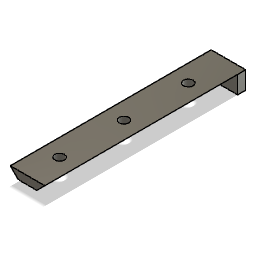
blind-joint-drill-guide-10mm-and-3z v3 (Autodesk Fusion 360 design; units mm, degrees)
Autodesk Fusion 360 part; units mm, degrees
sketch "Sketch1" plane through (0, 0, 0) normal (0, 0, 1) x (1, 0, 0)
  line L0 (-2.875, 0) -> (2.875, 0)
  line L1 (-5.375, 2.5) -> (5.375, 2.5)
  line L2 (-5.375, 2.5) -> (-2.875, 0)
  line L3 (5.375, 2.5) -> (2.875, 0)
  line L4 (0, 7.9451) -> (0, -6.0549)
  dimension "d1" = 5.75
  dimension "d2" = 10.75
  dimension "d3" = 2.5
  constraint horizontal L0
  constraint horizontal L1
  constraint vertical L4
  constraint symmetric L1.start L1.end L4
  constraint symmetric L0.start L0.end L4
  constraint vertical origin L4.end
  constraint horizontal origin L0.start
  measures "d1" distance of L0.start L0.end
  measures "d2" distance of L1.start L1.end
  measures "d3" vertical distance of L0.start L1.start
extrude "Extrude1" add sketch "Sketch1" along normal blind 60
sketch "Sketch2" plane through (0, 0, 0) normal (0, 0, -1) x (-1, 0, 0)
  line L0 (2.875, 0) -> (5.375, 2.5)
  line L1 (5.375, 2.5) -> (-5.375, 2.5)
  line L2 (-5.375, 2.5) -> (-2.875, 0)
  line L3 (-2.875, 0) -> (2.875, 0)
  line L4 (-5.375, 2.5) -> (5.375, 2.5)
  line L5 (5.375, 2.5) -> (5.375, -3)
  line L6 (5.375, -3) -> (-5.375, -3)
  line L7 (-5.375, -3) -> (-5.375, 2.5)
  dimension "d6" = 10.75
  dimension "d7" = 5.5
  constraint horizontal L4
  constraint vertical L5
  constraint horizontal L6
  constraint vertical L7
  constraint coincident L1.end L2.start
  measures "d6" distance of L1.end L0.end
  measures "d7" distance of L1.end L6.end
extrude "Extrude2" add sketch "Sketch2" along normal blind 2.5
sketch "Sketch3" plane through (0, 0, 0) normal (0, -1, 0) x (1, 0, 0)
  line L0 (-2.875, 0) -> (2.875, 0)
  line L1 (2.875, 0) -> (2.875, 60)
  line L2 (2.875, 60) -> (-2.875, 60)
  line L3 (-2.875, 60) -> (-2.875, 0)
  circle A0 centre (0, 10) radius 1.5
  circle A1 centre (0, 30) radius 1.5
  circle A2 centre (0, 50) radius 1.5
  dimension "d10" = 3
  dimension "d11" = 10
  dimension "d12" = 30
  dimension "d13" = 20
  constraint equal A1 A2
  constraint equal A0 A1
  measures "d10" diameter of A0
  measures "d11" distance of origin A0.centre
  measures "d12" distance of origin A1.centre
  measures "d13" distance of A1.centre A2.centre
extrude "Extrude3" cut sketch "Sketch3" against normal through all contours A0 | A1 | A2
